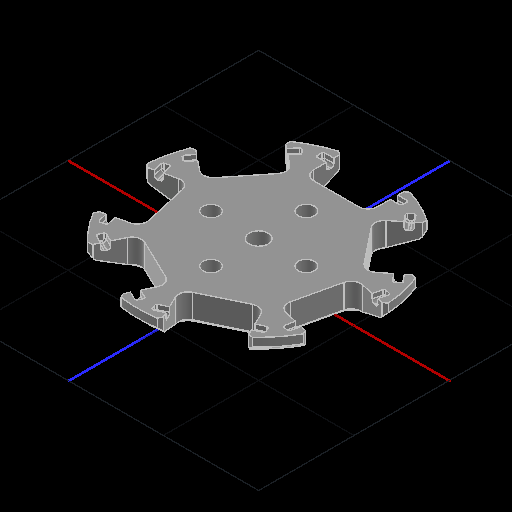
# Autodesk Inventor part: 2.75 inner
Saved by Autodesk Inventor 2025.2 (Build 292293000, 293)
## iProperties
Created: 2025-11-15
Part Number: 2.75 inner
Material: white pla
Document SubType Name: Modeling
Designer: cloudy
Density: 1 g/cm^3
Appearance: Smooth - Dark Gray
Author: cloudy
Autodesk Inventor part; units mm, degrees
ref_plane "YZ Plane" through (0, 0, 0) normal (1, 0, 0) x (0, 1, 0)
ref_plane "XZ Plane" through (0, 0, 0) normal (0, 1, 0) x (-1, 0, 0)
ref_plane "XY Plane" through (0, 0, 0) normal (0, 0, 1) x (1, 0, 0)
sketch "Sketch1" plane through (0, 0, 0) normal (0, 1, 0) x (-1, 0, 0)
  circle A0 centre (0, 0) radius 34.29
  dimension "d0" = 68.58
  constraints: 1 centre point, 1 coincident
  measures "d0" diameter of A0
extrude "Main Body Extrusion" add sketch "Sketch1" along normal blind 7.35
sketch "Main Sketch" plane through (0, 7.35, 0) normal (0, 1, 0) x (1, 0, 0)
  circle A0 centre (0, 0) radius 34.29 construction
  line L0 (0, 0) -> (0, 34.29) construction
  line L1 (-8.3, 34.29) -> (8.3, 34.29) construction
  line L2 (8.3, 34.29) -> (8.3, 20.865) construction
  line L3 (8.3, 20.865) -> (-8.3, 20.865) construction
  line L4 (-8.3, 20.865) -> (-8.3, 34.29) construction
  line L5 (-8.3, 34.29) -> (8.3, 20.865) construction
  line L6 (8.3, 34.29) -> (-8.3, 20.865) construction
  line L7 (8.5, 34.6203) -> (8.5, 20.665)
  line L8 (8.5, 20.665) -> (-8.5473, 20.665)
  line L9 (-8.5473, 20.665) -> (-8.5473, 34.6203)
  line L10 (-11.35, 28.5775) -> (11.35, 28.5775)
  line L11 (11.35, 28.5775) -> (11.35, 26.5775)
  line L12 (11.35, 26.5775) -> (-11.35, 26.5775)
  line L13 (-11.35, 26.5775) -> (-11.35, 28.5775)
  line L14 (-11.35, 28.5775) -> (11.35, 26.5775) construction
  line L15 (11.35, 28.5775) -> (-11.35, 26.5775) construction
  circle A1 centre (0, 0) radius 32.2489
  circle A2 centre (0, 0) radius 38.1
  line L16 (-11.35, 28.5775) -> (-11.9037, 29.9716) construction
  point P0 (0, 27.5775)
  point P1 (8.5, 31.1086)
  point P2 (-8.5473, 31.0956)
  dimension "d3" = 13.425
  dimension "d4" = 16.6
  dimension "d5" = 0.2
  dimension "d6" = 0.2
  dimension "d7" = 22.7
  dimension "d8" = 2
  dimension "d9" = 76.2
  dimension "d10" = 1.5
  constraints: 34 end point, 5 parallel, 4 midpoint, 3 horizontal, 2 coincident, 2 perpendicular, 2 point on line, 1 centre point, 1 vertical, 1 vertical alignment, 5 other
  measures "d3" distance of L1.end L2.end
  measures "d4" distance of L2.end L3.end
  measures "d5" distance between parallel lines of L2 L7
  measures "d6" distance between parallel lines of L3 L8
  measures "d7" distance of L11.end L12.end
  measures "d8" distance of L12.end L10.start
  measures "d9" diameter of A2
  measures "d10" distance of L10.start L16.end
extrude "Extrusion2" cut sketch "Main Sketch" against normal through all
extrude "Extrusion3" cut sketch "Main Sketch" against normal blind 2 contours L10 L11 L12 L7 | L7 L12 L9 L10 | L9 L12 L13 L10
extrude "Extrusion4" cut sketch "Main Sketch" against normal through all contours L7 L10 L9 A1 | L7 L12 L9 L10 | L7 L8 L9 L12
fillet "Fillet1" radius 2.54 2 edges at (-8.5473, 3.675, -20.665) (8.5, 3.675, -20.665)
chamfer "Chamfer1" distance 5.08 angle 45 1 edges at (0.0245, 0, 32.2489)
chamfer "Chamfer2" distance 5.08 angle 45 1 edges at (0.0249, 0, 27.1689)
chamfer "Chamfer3" distance 1 angle 45 5 edges at (6.5338, 0, -20.7307) (-0.0236, 0, -20.665) (-6.5705, 0, -20.7282) (8.5, 6.215, -31.1086) (-8.5473, 6.215, -31.0956)
fillet "Fillet2" radius 0.75 4 edges at (-9.9486, 5.35, -26.5775) (9.925, 5.35, -26.5775) (9.925, 5.35, -28.5775) (-9.9486, 5.35, -28.5775)
chamfer "Chamfer4" distance 0.35 angle 45 10 edges at (-11.35, 6.725, -28.5775) (-11.35, 5.5697, -28.3578) (-11.35, 5.35, -27.5775) (-11.35, 5.5697, -26.7972) (-11.35, 6.725, -26.5775) (11.35, 5.5697, -28.3578) (11.35, 5.35, -27.5775) (11.35, 5.5697, -26.7972) (11.35, 6.725, -26.5775) (11.35, 6.725, -28.5775)
pattern_circular "Circular Pattern1" count 7 over 360 about axis through (0, 7.35, 0) along (0, -1, 0) of "Extrusion4", "Fillet2", "Extrusion3", "Chamfer4", "Fillet1", "Chamfer3"
sketch "Sketch3" plane through (0, 0, 0) normal (0, -1, 0) x (1, 0, 0)
  circle A0 centre (0, 0) radius 2.54
  dimension "d34" = 5.08
  constraints: 1 centre point, 1 coincident
  measures "d34" diameter of A0
extrude "Extrusion5" cut sketch "Sketch3" against normal through all
sketch "Sketch4" plane through (0, 7.35, 0) normal (0, 1, 0) x (1, 0, 0)
  circle A0 centre (0, 12.7) radius 2.1844
  line L0 (0, 0) -> (0, 12.7) construction
  dimension "d37" = 4.3688
  dimension "d38" = 12.7
  constraints: 2 end point, 1 centre point, 1 vertical
  measures "d37" diameter of A0
  measures "d38" distance of L0.start L0.end
extrude "Extrusion6" cut sketch "Sketch4" against normal through all
pattern_circular "Circular Pattern2" count 4 over 360 about axis through (0, 0, 0) along (0, 1, 0) of "Extrusion6"
equation "\"d6\" = d5"
body "Solid1"
